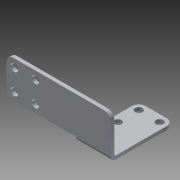
# Autodesk Inventor part: V5 Conveyor Plate Bracket P1 (45 deg)
Saved by Autodesk Inventor 2014 SP1 (Build 180222100, 222)
## iProperties
Created: 2012-03-30
Part Number: V5 Conveyor Plate Bracket P1 (45 deg)
Material: Aluminum-6061
Document SubType Name: Sheet Metal
Designer: Moses
Mass: 40.6749 g
Surface Area: 110.648 cm^2
Volume: 15.0092 cm^3
Density: 2.71 g/cm^3
Sheet Metal Rule: Default
Appearance: Aluminum - Flat
Author: Moses
Autodesk Inventor part; units mm, degrees
ref_plane "YZ Plane" through (0, 0, 0) normal (1, 0, 0) x (0, 1, 0)
ref_plane "XZ Plane" through (0, 0, 0) normal (0, 1, 0) x (-1, 0, 0)
ref_plane "XY Plane" through (0, 0, 0) normal (0, 0, 1) x (1, 0, 0)
sketch "Sketch1" plane through (0, 0, 0) normal (0, 0, 1) x (1, 0, 0)
  arc A0 (-6.35, -27.305) -> (0, -33.655) centre (0, -27.305) ccw
  line L0 (0, -33.655) -> (57.15, -33.655)
  line L1 (57.15, -33.655) -> (57.15, -84.1993)
  arc A1 (57.15, -84.1993) -> (63.5, -90.5493) centre (63.5, -84.1993) ccw
  line L2 (63.5, -90.5493) -> (82.55, -90.5493)
  arc A2 (82.55, -90.5493) -> (88.9, -84.1993) centre (82.55, -84.1993) ccw
  line L3 (88.9, -84.1993) -> (88.9, -6.35)
  arc A3 (88.9, -6.35) -> (82.55, 0) centre (82.55, -6.35) ccw
  line L4 (82.55, 0) -> (0, 0)
  arc A4 (0, 0) -> (-6.35, -6.35) centre (0, -6.35) ccw
  line L5 (-6.35, -6.35) -> (-6.35, -27.305)
  circle A5 centre (20.0025, -7.3025) radius 3.3782
  circle A6 centre (20.0025, -26.3525) radius 3.3782
  circle A7 centre (0.9525, -7.3025) radius 3.3782
  circle A8 centre (0.9525, -26.3525) radius 3.3782
  circle A9 centre (63.5, -65.1493) radius 3.3782
  circle A10 centre (82.55, -84.1993) radius 3.3782
  circle A11 centre (63.5, -84.1993) radius 3.3782
  line L6 (57.15, -35.7497) -> (88.9, -35.7497) construction
  line L7 (0.9525, -7.3025) -> (20.0025, -7.3025) construction
  line L8 (0.9525, -7.3025) -> (0.9525, -26.3525) construction
  line L9 (0.9525, -26.3525) -> (20.0025, -26.3525) construction
  line L10 (63.5, -65.1493) -> (63.5, -84.1993) construction
  line L11 (63.5, -84.1993) -> (82.55, -84.1993) construction
  dimension "d0" = 6.35
  dimension "d1" = 33.655
  dimension "d2" = 31.75
  dimension "d3" = 19.05
  dimension "d4" = 19.05
  dimension "d5" = 19.05
  dimension "d6" = 19.05
  dimension "d7" = 6.7564
  dimension "d8" = 6.7564
  dimension "d9" = 35.7497
  dimension "d10" = 95.25
  dimension "d11" = 90.5493
  dimension "d12" = 7.3025
  dimension "d13" = 7.3025
  dimension "d14" = 6.35
  dimension "d15" = 6.35
  dimension "d16" = 19.05
  constraints: 24 end point, 12 centre point, 10 point on circle, 10 tangent, 9 equal radius, 5 perpendicular, 2 point on line, 1 coincident, 1 horizontal, 1 parallel
  measures "d0" radius of A4
  measures "d1" distance between parallel lines of L4 L0
  measures "d2" distance between parallel lines of L3 L1
  measures "d3" distance of L7.end L7.start
  measures "d4" distance of L8.end L7.start
  measures "d5" distance of L10.end L10.start
  measures "d6" distance of A1.centre L11.end
  measures "d7" diameter of A9
  measures "d8" diameter of A7
  measures "d9" distance between parallel lines of L4 L6
  measures "d10" distance between parallel lines of L5 L3
  measures "d11" distance between parallel lines of L2 L4
  measures "d12" distance between parallel lines of L8 L5
  measures "d13" distance between parallel lines of L4 L7
  measures "d14" distance between parallel lines of L10 L1
  measures "d15" distance between parallel lines of L2 L11
  measures "d16" distance of L8.end L9.end
extrude "Plate1" add sketch "Sketch1" along normal blind 3.175
fold "Fold1" angle 90 bend radius 1.27 thickness 3.175 k factor 0.44 line from (57.15, -35.7497, 0) to (88.9, -35.7497, 0) line at bend centre moving side (0, -1, 0) folds toward (0, 0, -1)
equation "\"d18\" = BendReliefWidth"
equation "\"d19\" = BendReliefDepth"
equation "\"d20\" = MinimumRemnant"
equation "\"d21\" = BendRadius"
equation "\"BendRadius\" = Thickness"
equation "\"BendReliefWidth\" = Thickness"
equation "\"BendReliefDepth\" = 0.5 * Thickness"
equation "\"CornerReliefSize\" = 4 * Thickness"
equation "\"MinimumRemnant\" = 2 * Thickness"
equation "\"TransitionRadius\" = BendRadius"
equation "\"JacobiRadiusSize\" = BendRadius"
equation "\"GapSize\" = Thickness"
equation "\"d17\" = BendRadius"
equation "\"Thickness\" = 3.175"
body "Solid1"
